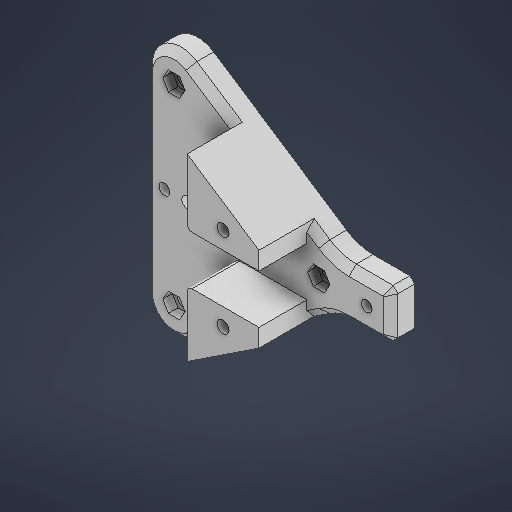
# Autodesk Inventor part: y axis something back
Saved by Autodesk Inventor 2026 (Build 300175000, 175)
## iProperties
Created: 2025-02-02
Part Number: y axis something back
Material: Generic
Document SubType Name: Modeling
Designer: jerem
Density: 1 g/cm^3
Appearance: Default
Author: jerem
## iProperties of the stored document y axis something back_3DPrint.ipt
Created: 2025-02-19
Part Number: y axis something back_3DPrint
Material: Generic
Document SubType Name: Modeling
Designer: jerem
Density: 1 g/cm^3
Appearance: Default
Author: jerem
Autodesk Inventor part; units mm, degrees
ref_plane "YZ Plane" through (0, 0, 0) normal (1, 0, 0) x (0, 1, 0)
ref_plane "XZ Plane" through (0, 0, 0) normal (0, 1, 0) x (-1, 0, 0)
ref_plane "XY Plane" through (0, 0, 0) normal (0, 0, 1) x (1, 0, 0)
sketch "Sketch1" plane through (0, 0, 0) normal (0, 0, 1) x (1, 0, 0)
  line L0 (0, 0) -> (30.25, 0) construction
  line L1 (0, 0) -> (-30.25, 0) construction
  line L2 (-30.25, 0) -> (-30.25, 40) construction
  line L3 (-30.25, 0) -> (-30.25, -40) construction
  circle A0 centre (-30.25, 40) radius 2.7
  circle A1 centre (-30.25, -40) radius 2.7
  circle A2 centre (30.25, 0) radius 2.7
  circle A3 centre (-30.25, 40) radius 12
  circle A4 centre (-30.25, -40) radius 12
  circle A5 centre (30.25, 0) radius 12
  line L4 (36.868172, -10.009985) -> (-23.631828, -50.009985)
  line L5 (-42.25, 40) -> (-42.25, -40)
  circle A6 centre (-34.25, 0) radius 2.25
  line L6 (-30.25, 0) -> (-34.25, 0) construction
  line L7 (-23.631828, 50.009985) -> (36.868172, 10.009985)
  line L8 (30.25, 0) -> (50.25, 0) construction
  circle A7 centre (50.25, 0) radius 10
  circle A8 centre (50.25, 0) radius 2.25
  line L9 (50.25746, 9.999997) -> (36.868172, 10.009985)
  line L10 (50.25746, -9.999997) -> (36.868172, -10.009985)
  circle A9 centre (10.25, 0) radius 2.25
  line L11 (50.25746, -9.999997) -> (60.257457, -9.992538)
  line L12 (60.257457, -9.992538) -> (60.242549, 9.992549)
  line L13 (60.242549, 9.992549) -> (50.25746, 9.999997)
  point P0 (-42.25, 0)
  point P1 (41.35, -4.559605)
  point P2 (41.35, 4.559605)
  point P3 (60.249997, 0.00746)
  dimension "d0" = 60.5
  dimension "d1" = 5.4
  dimension "d2" = 80
  dimension "d3" = 24
  dimension "d55" = 4.5
  dimension "d56" = 8
  dimension "d57" = 20
  dimension "d58" = 20
  dimension "d69" = 20
  constraints: 28 end point, 10 centre point, 10 tangent, 8 coincident, 8 point on circle, 6 equal radius, 4 horizontal, 2 collinear, 2 perpendicular, 2 vertical, 1 midpoint, 1 point on line
  measures "d0" distance of L0.end L1.end
  measures "d1" diameter of A0
  measures "d2" distance of L3.end L2.end
  measures "d3" diameter of A3
  measures "d55" diameter of A6
  measures "d56" distance of point (-42.25, 0) L6.end
  measures "d57" distance of L8.start L8.end
  measures "d58" diameter of A7
  measures "d69" distance of A9.centre L0.end
sketch "Sketch1 outline for Extrusion1" plane through (0, 0, 0) normal (0, 0, 1) x (1, 0, 0)
  arc A0 (-23.631828, 50.009985) -> (-42.25, 40) centre (-30.25, 40) ccw
  line L0 (-42.25, 40) -> (-42.25, -40)
  arc A1 (-42.25, -40) -> (-23.631828, -50.009985) centre (-30.25, -40) ccw
  line L1 (-23.631828, -50.009985) -> (36.868172, -10.009985)
  line L2 (36.868172, -10.009985) -> (60.257457, -9.992538)
  line L3 (60.257457, -9.992538) -> (60.242549, 9.992549)
  line L4 (60.242549, 9.992549) -> (36.868172, 10.009985)
  line L5 (36.868172, 10.009985) -> (-23.631828, 50.009985)
  circle A2 centre (-30.25, 40) radius 2.7
  circle A3 centre (10.25, 0) radius 2.25
  circle A4 centre (-34.25, 0) radius 2.25
  circle A5 centre (30.25, 0) radius 2.7
  circle A6 centre (-30.25, -40) radius 2.7
  circle A7 centre (50.25, 0) radius 2.25
extrude "Extrusion1" add sketch "Sketch1 outline for Extrusion1" against normal blind 10
fillet "Fillet1" radius 20 2 edges at (36.8682, 10.01, -5) (36.8682, -10.01, -5)
chamfer "Chamfer6" distance 2 angle 45 2 edges at (60.2425, 9.9925, -5) (60.2575, -9.9925, -5)
sketch "Sketch8" plane through (0, 0, 0) normal (0, 0, 1) x (1, 0, 0)
  line L0 (58.257457, -9.99403) -> (60.255965, -7.992538)
  line L1 (58.257457, -9.99403) -> (42.873828, -10.005505)
  arc A0 (42.873828, -10.005505) -> (31.85846, -13.322191) centre (42.888747, -30.0055) ccw
  line L2 (31.85846, -13.322191) -> (-23.631828, -50.009985)
  arc A1 (-42.25, -40) -> (-23.631828, -50.009985) centre (-30.25, -40) ccw
  line L3 (-42.25, -40) -> (-42.25, 40)
  arc A2 (-23.631828, 50.009985) -> (-42.25, 40) centre (-30.25, 40) ccw
  line L4 (-23.631828, 50.009985) -> (31.85846, 13.322191)
  arc A3 (31.85846, 13.322191) -> (42.873828, 10.005505) centre (42.888747, 30.0055) ccw
  line L5 (42.873828, 10.005505) -> (58.242549, 9.994041)
  line L6 (60.244041, 7.992549) -> (58.242549, 9.994041)
  line L7 (60.244041, 7.992549) -> (60.255965, -7.992538)
  circle A4 centre (30.25, 0) radius 2.7
  circle A5 centre (50.25, 0) radius 2.25
  circle A6 centre (-30.25, -40) radius 2.7
  circle A7 centre (-34.25, 0) radius 2.25
  circle A8 centre (10.25, 0) radius 2.25
  circle A9 centre (-30.25, 40) radius 2.7
  line L8 (-27.926165, -44.025) -> (-32.573835, -44.025)
  line L9 (-32.573835, -44.025) -> (-34.89767, -40)
  line L10 (-34.89767, -40) -> (-32.573835, -35.975)
  line L11 (-32.573835, -35.975) -> (-27.926165, -35.975)
  line L12 (-27.926165, -35.975) -> (-25.60233, -40)
  line L13 (-25.60233, -40) -> (-27.926165, -44.025)
  line L14 (-27.926165, 35.975) -> (-32.573835, 35.975)
  line L15 (-32.573835, 35.975) -> (-34.89767, 40)
  line L16 (-34.89767, 40) -> (-32.573835, 44.025)
  line L17 (-32.573835, 44.025) -> (-27.926165, 44.025)
  line L18 (-27.926165, 44.025) -> (-25.60233, 40)
  line L19 (-25.60233, 40) -> (-27.926165, 35.975)
  line L20 (32.573835, -4.025) -> (27.926165, -4.025)
  line L21 (27.926165, -4.025) -> (25.60233, 0)
  line L22 (25.60233, 0) -> (27.926165, 4.025)
  line L23 (27.926165, 4.025) -> (32.573835, 4.025)
  line L24 (32.573835, 4.025) -> (34.89767, 0)
  line L25 (34.89767, 0) -> (32.573835, -4.025)
  point P0 (0, 0)
  dimension "d83" = 8.05
  dimension "d84" = 8.05
  dimension "d85" = 8.05
  constraints: 36 end point, 3 coincident, 3 horizontal, 39 other
  measures "d83" distance between parallel lines of L23 L20
  measures "d84" distance between parallel lines of L17 L14
  measures "d85" distance between parallel lines of L11 L8
extrude "Extrusion9" cut sketch "Sketch8" against normal blind 4 contours L8 L9 L10 L11 L12 L13 | L14 L15 L16 L17 L18 L19 | L20 L21 L22 L23 L24 L25
sketch "Sketch5" plane through (0, 0, 0) normal (0, 0, 1) x (1, 0, 0)
  arc A0 (-42.25, -40) -> (-23.631828, -50.009985) centre (-30.25, -40) ccw
  line L0 (-23.631828, -50.009985) -> (31.85846, -13.322191)
  arc A1 (42.873828, -10.005505) -> (31.85846, -13.322191) centre (42.888747, -30.0055) ccw
  line L1 (42.873828, -10.005505) -> (58.257457, -9.99403)
  arc A2 (31.85846, 13.322191) -> (42.873828, 10.005505) centre (42.888747, 30.0055) ccw
  line L2 (31.85846, 13.322191) -> (-23.631828, 50.009985)
  arc A3 (-23.631828, 50.009985) -> (-42.25, 40) centre (-30.25, 40) ccw
  line L3 (-42.25, 40) -> (-42.25, -40)
  circle A4 centre (-34.25, 0) radius 2.25
  circle A5 centre (50.25, 0) radius 2.25
  line L4 (-4.75, 10.2) -> (-4.75, 37.526132)
  line L5 (-4.75, 10.2) -> (25.25, 10.2)
  line L6 (25.25, 10.2) -> (25.25, 17.691421)
  line L7 (60.255965, -7.992538) -> (60.244041, 7.992549)
  line L8 (58.242549, 9.994041) -> (42.873828, 10.005505)
  line L9 (60.255965, -7.992538) -> (58.257457, -9.99403)
  line L10 (58.242549, 9.994041) -> (60.244041, 7.992549)
  dimension "d66" = 30
  dimension "d92" = 10.2
  dimension "d93" = 25
  constraints: 6 end point, 2 point on line, 1 horizontal, 1 perpendicular, 1 vertical, 1 other
  measures "d66" distance of L4.start L5.end
  measures "d92" distance from line of L5 A5.centre
  measures "d93" distance from line of A5.centre L6
extrude "Extrusion6" add sketch "Sketch5" along normal blind 20 contours L2 L6 L5 L4
sketch "Sketch9" plane through (0, 0, 20) normal (0, 0, 1) x (1, 0, 0)
  circle A0 centre (10.25, 0) radius 2.25
  line L0 (25.25, 10.2) -> (25.25, 17.691421)
  line L1 (25.25, 17.691421) -> (-4.75, 37.526132)
  line L2 (-4.75, 37.526132) -> (-4.75, 10.2)
  line L3 (-4.75, 10.2) -> (25.25, 10.2)
  line L4 (10.25, 0) -> (10.25, 17.5) construction
  circle A1 centre (10.25, 17.5) radius 2.5
  point P0 (0, 0)
  dimension "d88" = 17.5
  dimension "d89" = 5
  constraints: 2 end point, 1 centre point, 1 coincident, 1 vertical
  measures "d88" distance of L4.start L4.end
  measures "d89" diameter of A1
extrude "Extrusion10" cut sketch "Sketch9" against normal blind 5 contours A1
mirror "Mirror1" about plane through (0, 0, 0) normal (0, 1, 0) of "Extrusion10", "Extrusion6"
fillet "Fillet2" radius 2 2 edges at (-4.75, 10.2, 10) (-4.75, -10.2, 10)
sketch "Sketch10" plane through (0, 0, -10) normal (0, 0, -1) x (-1, 0, 0)
  circle A0 centre (-50.25, 0) radius 2.25 projected
  circle A1 centre (-10.25, 0) radius 2.25 projected
  circle A2 centre (-50.25, 0) radius 4
  circle A3 centre (-10.25, 0) radius 4
  point P0 (0, 0)
  dimension "d95" = 8
  constraints: 2 centre point, 2 coincident, 1 equal radius
  measures "d95" diameter of A2
extrude "Extrusion11" cut sketch "Sketch10" against normal blind 5 contours A0 | A1 | A2 | A3
sketch "Sketch11" plane through (0, 0, 0) normal (0, 0, 1) x (1, 0, 0)
  arc A0 (-4.75, 12.2) -> (-2.75, 10.2) centre (-2.75, 12.2) ccw
  line L0 (-2.75, 10.2) -> (25.25, 10.2)
  line L1 (25.25, 10.2) -> (25.25, 17.691421)
  line L2 (25.25, 17.691421) -> (-4.75, 37.526132)
  line L3 (-4.75, 37.526132) -> (-4.75, 12.2)
  circle A1 centre (10.25, 17.5) radius 2.5
  arc A2 (-2.75, -10.2) -> (-4.75, -12.2) centre (-2.75, -12.2) ccw
  line L4 (-4.75, -37.526132) -> (-4.75, -12.2)
  line L5 (25.25, -17.691421) -> (-4.75, -37.526132)
  line L6 (25.25, -10.2) -> (25.25, -17.691421)
  line L7 (-2.75, -10.2) -> (25.25, -10.2)
  circle A3 centre (10.25, -17.5) radius 2.5
  line L8 (25.25, -10.2) -> (25.25, -17.691421)
  line L9 (25.25, -17.691421) -> (31.85846, -13.322191)
  arc A4 (42.873828, -10.005505) -> (31.85846, -13.322191) centre (42.888747, -30.0055) ccw
  line L10 (42.873828, -10.005505) -> (58.257457, -9.99403)
  line L11 (60.255965, -7.992538) -> (58.257457, -9.99403)
  line L12 (60.255965, -7.992538) -> (60.244041, 7.992549)
  line L13 (58.242549, 9.994041) -> (60.244041, 7.992549)
  line L14 (58.242549, 9.994041) -> (42.873828, 10.005505)
  arc A5 (31.85846, 13.322191) -> (42.873828, 10.005505) centre (42.888747, 30.0055) ccw
  line L15 (31.85846, 13.322191) -> (25.25, 17.691421)
  line L16 (25.25, 17.691421) -> (25.25, 10.2)
  line L17 (25.25, 10.2) -> (-2.75, 10.2)
  arc A6 (-4.75, 12.2) -> (-2.75, 10.2) centre (-2.75, 12.2) ccw
  line L18 (-4.75, 12.2) -> (-4.75, 37.526132)
  line L19 (-4.75, 37.526132) -> (-23.631828, 50.009985)
  arc A7 (-23.631828, 50.009985) -> (-42.25, 40) centre (-30.25, 40) ccw
  line L20 (-42.25, 40) -> (-42.25, -40)
  arc A8 (-42.25, -40) -> (-23.631828, -50.009985) centre (-30.25, -40) ccw
  line L21 (-23.631828, -50.009985) -> (-4.75, -37.526132)
  line L22 (-4.75, -37.526132) -> (-4.75, -12.2)
  arc A9 (-2.75, -10.2) -> (-4.75, -12.2) centre (-2.75, -12.2) ccw
  line L23 (-2.75, -10.2) -> (25.25, -10.2)
  line L24 (-32.573835, 44.025) -> (-27.926165, 44.025)
  line L25 (-27.926165, 44.025) -> (-25.60233, 40)
  line L26 (-25.60233, 40) -> (-27.926165, 35.975)
  line L27 (-27.926165, 35.975) -> (-32.573835, 35.975)
  line L28 (-32.573835, 35.975) -> (-34.89767, 40)
  line L29 (-34.89767, 40) -> (-32.573835, 44.025)
  line L30 (-32.573835, -35.975) -> (-27.926165, -35.975)
  line L31 (-27.926165, -35.975) -> (-25.60233, -40)
  line L32 (-25.60233, -40) -> (-27.926165, -44.025)
  line L33 (-27.926165, -44.025) -> (-32.573835, -44.025)
  line L34 (-32.573835, -44.025) -> (-34.89767, -40)
  line L35 (-34.89767, -40) -> (-32.573835, -35.975)
  line L36 (27.926165, 4.025) -> (32.573835, 4.025)
  line L37 (32.573835, 4.025) -> (34.89767, 0)
  line L38 (34.89767, 0) -> (32.573835, -4.025)
  line L39 (32.573835, -4.025) -> (27.926165, -4.025)
  line L40 (27.926165, -4.025) -> (25.60233, 0)
  line L41 (25.60233, 0) -> (27.926165, 4.025)
  circle A10 centre (50.25, 0) radius 2.25
  circle A11 centre (-34.25, 0) radius 2.25
  circle A12 centre (10.25, 0) radius 2.25
  line L42 (-4.75, 12.2) -> (-4.75, -12.2)
  circle A13 centre (-4.75, 0) radius 2.25
  circle A14 centre (-24.75, 0) radius 2.25
  line L43 (-24.75, 2.25) -> (-4.75, 2.25)
  line L44 (-4.75, -2.25) -> (-24.75, -2.25)
  line L45 (-24.75, 0) -> (-4.75, 0) construction
  line L46 (-4.75, 0) -> (-4.75, 0)
  line L47 (0, 0) -> (-4.75, 0) construction
  dimension "d98" = 4.5
  dimension "d100" = 20
  constraints: 12 end point, 5 tangent, 4 point on circle, 2 centre point, 2 horizontal, 1 collinear, 1 equal radius, 1 midpoint
  measures "d98" diameter of A14
  measures "d100" distance of L45.start L45.end
extrude "Extrusion12" cut sketch "Sketch11" against normal through all contours A13 L42 | L42 A13 | A13 L44 A14 L43 | A14
chamfer "Chamfer7" distance 3 angle 45 14 edges at (-14.1909, 43.7681, 0) (-35.9325, 50.5692, 0) (-42.25, 0, 0) (-35.9325, -50.5692, 0) (-14.1909, -43.7681, 0) (37.1225, 10.8548, 0) (50.5582, 9.9998, 0) (28.5542, 15.5068, 0) (60.25, 0, 0) (50.5656, -9.9998, 0) (37.1225, -10.8548, 0) (28.5542, -15.5068, 0) (59.2567, -8.9933, 0) (59.2433, 8.9933, 0)
equation "\"d84\" = d83"
equation "\"d85\" = d83"
equation "\"b\" = 2"
body "Solid1"
